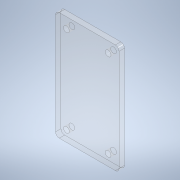
# Autodesk Inventor part: 103.017.01_Abdeckplatte_Extruderfuehrung
Saved by Autodesk Inventor 2021 (Build 250183000, 183)
## iProperties
Created: 2021-12-01
Part Number: 103.017.01_Abdeckplatte_Extruderfuehrung
Material: PMMA-Kunststoff
Document SubType Name: Modeling
Designer: Sebastian Seewald
Mass: 7.35751 g
Surface Area: 48.0913 cm^2
Volume: 6.19319 cm^3
Density: 1.188 g/cm^3
Appearance: Polycarbonat - klar
Author: Sebastian Seewald
Autodesk Inventor part; units mm, degrees
ref_plane "YZ Plane" through (0, 0, 0) normal (1, 0, 0) x (0, 1, 0)
ref_plane "XZ Plane" through (0, 0, 0) normal (0, 1, 0) x (-1, 0, 0)
ref_plane "XY Plane" through (0, 0, 0) normal (0, 0, 1) x (1, 0, 0)
sketch "Skizze1" plane through (0, 0, 0) normal (0, 0, 1) x (1, 0, 0)
  line L0 (2, 0) -> (33, 0)
  line L1 (35, 2) -> (35, 58)
  line L2 (33, 60) -> (2, 60)
  line L3 (0, 58) -> (0, 2)
  arc A0 (2, 60) -> (0, 58) centre (2, 58) ccw
  arc A1 (0, 2) -> (2, 0) centre (2, 2) ccw
  arc A2 (33, 0) -> (35, 2) centre (33, 2) ccw
  arc A3 (35, 58) -> (33, 60) centre (33, 58) ccw
  circle A4 centre (6, 54) radius 1.6
  circle A5 centre (29, 54) radius 1.6
  circle A6 centre (6, 6) radius 1.6
  circle A7 centre (29, 6) radius 1.6
  point P0 (0, 0)
  dimension "d0" = 60
  dimension "d1" = 35
  dimension "d2" = 2
  dimension "d3" = 3.2
  dimension "d4" = 3.2
  dimension "d5" = 3.2
  dimension "d6" = 3.2
  dimension "d7" = 6
  dimension "d8" = 6
  dimension "d9" = 6
  dimension "d10" = 6
  constraints: 8 centre point, 8 end point, 8 point on circle, 8 tangent, 3 equal radius, 2 horizontal alignment, 2 parallel, 2 point on line, 2 vertical alignment, 1 horizontal, 1 perpendicular
  measures "d0" distance between parallel lines of L0 L2
  measures "d1" distance between parallel lines of L3 L1
  measures "d2" radius of A0
  measures "d3" diameter of A4
  measures "d4" diameter of A5
  measures "d5" diameter of A7
  measures "d6" diameter of A6
  measures "d7" distance from line of L3 A4.centre
  measures "d8" distance from line of L2 A4.centre
  measures "d9" distance from line of L0 A6.centre
  measures "d10" distance from line of L1 A5.centre
extrude "Extrusion1" add sketch "Skizze1" along normal blind 3
